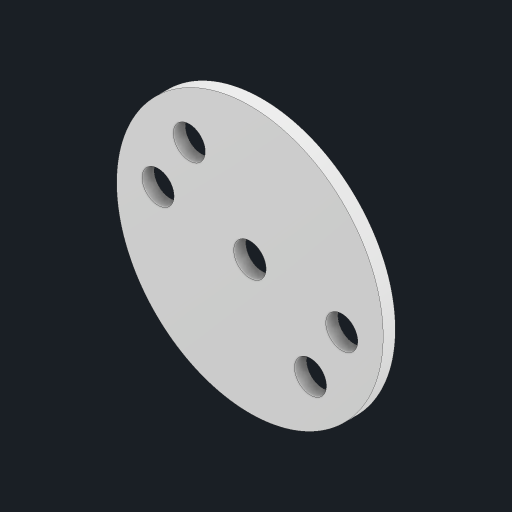
# Autodesk Inventor part: 2in_flex_wheel_hub
Saved by Autodesk Inventor 2024 (Build 280153000, 153)
## iProperties
Created: 2024-03-23
Part Number: 2in_flex_wheel_hub
Material: Acetal Resin, White
Document SubType Name: Modeling
Designer: Averey Ku
Density: 1.425 g/cm^3
Appearance: Smooth - White
Author: Averey Ku
Autodesk Inventor part; units mm, degrees
ref_plane "YZ Plane" through (0, 0, 0) normal (1, 0, 0) x (0, 1, 0)
ref_plane "XZ Plane" through (0, 0, 0) normal (0, 1, 0) x (-1, 0, 0)
ref_plane "XY Plane" through (0, 0, 0) normal (0, 0, 1) x (1, 0, 0)
sketch "main" plane through (0, 0, 0) normal (0, 0, 1) x (1, 0, 0)
  circle A0 centre (-3.5355, 3.6269) radius 17.4625
  arc A1 (-12.4711, 11.0953) -> (-10.1649, 11.3129) centre (-11.4711, 12.8274) ccw
  circle A2 centre (4.4001, -5.7121) radius 2.0955
  circle A3 centre (8.5065, 1.4036) radius 2.0955
  circle A4 centre (-11.482, 12.9439) radius 2.0955
  circle A5 centre (-15.5775, 5.8503) radius 2.0955
  circle A6 centre (-3.5355, 3.6269) radius 2.1209
  point P0 (-4.7735, 4.9064)
  point P1 (3.0939, -4.059)
  point P2 (5.4001, -3.8415)
  dimension "d0" = 4.191
  dimension "d1" = 34.925
  dimension "d2" = 4.191
  dimension "d3" = 4.191
  dimension "d4" = 4.191
  dimension "d5" = 4.2418
  measures "d0" diameter of A2
  measures "d1" diameter of A0
  measures "d2" diameter of A3
  measures "d3" diameter of A4
  measures "d4" diameter of A5
  measures "d5" diameter of A6
sketch "Sketch1" plane through (0, 0, 0) normal (0, 0, 1) x (1, 0, 0)
  circle A0 centre (0, 0) radius 17.4625
  arc A1 (-8.9356, 7.4684) -> (-6.6294, 7.686) centre (-7.9356, 9.2004) ccw
  circle A2 centre (7.9356, -9.3391) radius 2.0955
  circle A3 centre (12.042, -2.2234) radius 2.0955
  circle A4 centre (-7.9465, 9.317) radius 2.0955
  circle A5 centre (-12.042, 2.2234) radius 2.0955
  circle A6 centre (0, 0) radius 2.1209
  constraints: 1 other
extrude "Extrusion1" add sketch "Sketch1" along normal blind 1.5875 contours A0 | A4 A1
body "Solid1"
